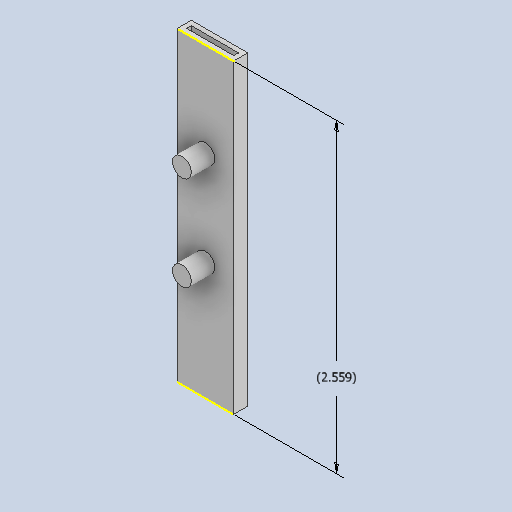
# Autodesk Inventor part: covet cover
Saved by Autodesk Inventor 2022 (Build 260153000, 153)
## iProperties
Created: 2022-08-26
Part Number: covet cover
Material: Generic
Document SubType Name: Modeling
Designer: yashm
Density: 1 g/cm^3
Appearance: Default
Author: yashm
Autodesk Inventor part; units mm, degrees
ref_plane "YZ Plane" through (0, 0, 0) normal (1, 0, 0) x (0, 1, 0)
ref_plane "XZ Plane" through (0, 0, 0) normal (0, 1, 0) x (-1, 0, 0)
ref_plane "XY Plane" through (0, 0, 0) normal (0, 0, 1) x (1, 0, 0)
sketch "Sketch1" plane through (0, 0, 0) normal (0, 0, 1) x (1, 0, 0)
  line L0 (0, 0) -> (12, 0)
  line L1 (12, 0) -> (12, 65)
  line L2 (12, 65) -> (0, 65)
  line L3 (0, 65) -> (0, 0)
  dimension "d0" = 65
  dimension "d1" = 12
  constraints: 8 end point, 2 parallel, 1 horizontal, 1 perpendicular
  measures "d0" distance of L0.end L1.end
  measures "d1" distance of L1.end L2.end
extrude "Extrusion1" add sketch "Sketch1" along normal blind 3
sketch "Sketch2" plane through (0, 0, 3) normal (0, 0, 1) x (1, 0, 0)
  circle A0 centre (6, 45) radius 2
  circle A1 centre (6, 25) radius 2
  line L0 (0, 65) -> (0, 0) projected
  line L1 (12, 0) -> (12, 65) projected
  line L2 (12, 65) -> (0, 65) projected
  dimension "d4" = 12
  dimension "d5" = 6
  dimension "d6" = 0
  dimension "d7" = 20
  dimension "d8" = 20
  dimension "d9" = 4
  constraints: 2 centre point, 1 equal radius
  measures "d4" distance between parallel lines of L0 L1
  measures "d5" distance from line of L1 A0.centre
  measures "d6" horizontal distance of A1.centre A0.centre
  measures "d7" distance from line of L2 A0.centre
  measures "d8" distance of A1.centre A0.centre
  measures "d9" diameter of A0
extrude "Extrusion2" add sketch "Sketch2" along normal blind 5
sketch "Sketch3" plane through (0, 65, 0) normal (0, 1, 0) x (1, 0, 0)
  line L0 (1, -2) -> (11, -2)
  line L1 (11, -2) -> (11, -1)
  line L2 (11, -1) -> (1, -1)
  line L3 (1, -1) -> (1, -2)
  line L4 (12, 0) -> (0, 0) projected
  line L5 (0, 0) -> (0, -3) projected
  line L6 (12, 0) -> (12, -3) projected
  dimension "d12" = 1
  dimension "d13" = 1
  dimension "d14" = 1
  dimension "d15" = 1
  constraints: 8 end point, 2 parallel, 1 horizontal, 1 perpendicular
  measures "d12" distance of L0.end L1.end
  measures "d13" distance between parallel lines of L4 L2
  measures "d14" distance between parallel lines of L5 L3
  measures "d15" distance between parallel lines of L1 L6
sketch "Sketch4" plane through (0, 0, 3) normal (0, 0, 1) x (1, 0, 0)
  line L0 (0, 0) -> (12, 0) projected
  line L1 (12, 65) -> (0, 65) projected
  dimension "d16" = 65
  measures "d16" distance between parallel lines of L0 L1
extrude "Extrusion3" cut sketch "Sketch3" against normal blind 63
sketch "Sketch5" plane through (0, 0, 0) normal (0, 0, -1) x (-1, 0, 0)
  point P0 (0, 0)
sketch "Sketch6" plane through (0, 0, 0) normal (0, 0, -1) x (-1, 0, 0)
  line L0 (-10, 61) -> (-2, 61)
  line L1 (-2, 61) -> (-2, 4)
  line L2 (-2, 4) -> (-10, 4)
  line L3 (-10, 4) -> (-10, 61)
  line L4 (0, 0) -> (-12, 0) projected
  line L5 (-12, 65) -> (0, 65) projected
  line L6 (0, 65) -> (0, 0) projected
  line L7 (-12, 0) -> (-12, 65) projected
  dimension "d19" = 4
  dimension "d20" = 4
  dimension "d21" = 2
  dimension "d22" = 2
  constraints: 8 end point, 2 parallel, 1 horizontal, 1 perpendicular
  measures "d19" distance between parallel lines of L4 L2
  measures "d20" distance between parallel lines of L5 L0
  measures "d21" distance between parallel lines of L6 L1
  measures "d22" distance between parallel lines of L7 L3
extrude "Extrusion4" cut sketch "Sketch6" against normal up to surface (2 mm away) contours L0 L1 L2 L3
body "Solid1"
